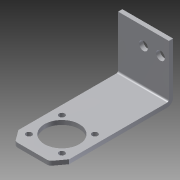
# Autodesk Inventor part: bracket for PG-71
Saved by Autodesk Inventor 2013 (Build 170138000, 138)
## iProperties
Created: 2013-02-02
Part Number: bracket for PG-71
Material: Aluminum 6061
Document SubType Name: Sheet Metal
Designer: aslane
Density: 1 g/cm^3
Sheet Metal Rule: Default
Author: aslane
Autodesk Inventor part; units mm, degrees
ref_plane "YZ Plane" through (0, 0, 0) normal (1, 0, 0) x (0, 1, 0)
ref_plane "XZ Plane" through (0, 0, 0) normal (0, 1, 0) x (-1, 0, 0)
ref_plane "XY Plane" through (0, 0, 0) normal (0, 0, 1) x (1, 0, 0)
sketch "Sketch1" plane through (0, 0, 0) normal (0, 1, 0) x (-1, 0, 0)
  line L0 (30.798, 43.1648) -> (0.6237, 2.4295)
  arc A0 (0.6237, 2.4295) -> (0, 0.5397) centre (3.175, 0.5397) ccw
  line L1 (0, 0.5397) -> (0, 0)
  line L2 (0, 0) -> (88.9, 0)
  line L3 (88.9, 0) -> (88.9, 0.5397)
  arc A1 (88.9, 0.5397) -> (88.2763, 2.4295) centre (85.725, 0.5397) ccw
  line L4 (88.2763, 2.4295) -> (58.102, 43.1648)
  arc A2 (58.102, 43.1648) -> (55.5507, 44.45) centre (55.5507, 41.275) ccw
  line L5 (55.5507, 44.45) -> (33.3493, 44.45)
  arc A3 (33.3493, 44.45) -> (30.798, 43.1648) centre (33.3493, 41.275) ccw
  circle A4 centre (15.875, 9.525) radius 4.7625
  circle A5 centre (44.45, 22.225) radius 13.0556
  circle A6 centre (56.8248, 34.5998) radius 2.1463
  circle A7 centre (56.8248, 9.8502) radius 2.1463
  circle A8 centre (32.0752, 9.8502) radius 2.1463
  circle A9 centre (32.0752, 34.5998) radius 2.1463
  circle A10 centre (73.025, 9.525) radius 4.7625
  line L6 (0, 0) -> (0, -42.1767)
  line L7 (0, -42.1767) -> (88.9, -42.1767)
  line L8 (88.9, -42.1767) -> (88.9, 0)
  dimension "d70" = 86.6267
  dimension "d71" = 3.175
  dimension "d72" = 9.525
  dimension "d73" = 4.2926
  dimension "d74" = 26.1112
  dimension "d75" = 143.471
  dimension "d76" = 90
  dimension "d77" = 36.529
  dimension "d78" = 90
  dimension "d79" = 88.9
  dimension "d80" = 44.45
  dimension "d81" = 88.9
  dimension "d82" = 72.3812
  dimension "d83" = 44.45
  dimension "d84" = 0.9449
  dimension "d85" = 15.875
  dimension "d86" = 8.0319
  dimension "d87" = 32.0752
  dimension "d88" = 6.1244
  dimension "d89" = 32.0752
  dimension "d90" = 20.8561
  dimension "d91" = 44.45
  dimension "d92" = 23.4341
  dimension "d93" = 56.8248
  dimension "d94" = 26.0121
  dimension "d95" = 56.8248
  dimension "d96" = 40.7438
  dimension "d97" = 73.025
  dimension "d98" = 53.9552
  measures "d70" distance between parallel lines of L7 L5
  measures "d71" radius of A1
  measures "d72" diameter of A10
  measures "d73" diameter of A6
  measures "d74" diameter of A5
  measures "d75" angle of L3 L4
  measures "d76" angle of L3 L5
  measures "d77" angle of L3 L0
  measures "d78" angle of L5 L1
  measures "d79" distance between parallel lines of L8 L6
  measures "d80" distance between parallel lines of L2 L5
  measures "d81" distance from line of point (0, 0) L3
  measures "d82" distance from line of point (0, 0) L4
  measures "d83" distance from line of point (0, 0) L5
  measures "d84" distance from line of point (0, 0) L0
  measures "d85" distance from line of A10.centre L3
  measures "d86" distance from line of A10.centre L4
  measures "d87" distance from line of A6.centre L3
  measures "d88" distance from line of A6.centre L4
  measures "d89" distance from line of A7.centre L3
  measures "d90" distance from line of A7.centre L4
  measures "d91" distance from line of A5.centre L3
  measures "d92" distance from line of A5.centre L4
  measures "d93" distance from line of A9.centre L3
  measures "d94" distance from line of A9.centre L4
  measures "d95" distance from line of A8.centre L3
  measures "d96" distance from line of A8.centre L4
  measures "d97" distance from line of A4.centre L3
  measures "d98" distance from line of A4.centre L4
extrude "Plate1" add sketch "Sketch1" along normal blind 3.175
sketch "Sketch9" plane through (-88.9, 0, -39.0017) normal (0, 0, -1) x (-1, 0, 0)
  line L0 (-88.9, 0) -> (0, 0)
  line L1 (0, 0) -> (0, 37.465)
  line L2 (0, 37.465) -> (-88.9, 37.465)
  line L3 (-88.9, 37.465) -> (-88.9, 0)
  constraints: 6 end point, 1 horizontal, 1 perpendicular, 1 vertical
edge flange "Flange2" height 37.465 angle 90 thickness 3.175 bend radius 1.27 thickness toward (0, 0, -1) relief straight relief width 3.175 relief depth 1.5875 edges at (-44.45, 3.175, -42.1767) wall of the first edge with corners at (0, 0, -39.0017) (-88.9, 0, -39.0017) (-88.9, 37.465, -39.0017) (0, 37.465, -39.0017)
bend "Bend5"
corner "Corner2"
sketch "Sketch10" plane through (-88.9, 37.465, -42.1767) normal (0, 1, 0) x (1, 0, 0)
  line L0 (88.9, 0) -> (0, 0) projected
  line L1 (0, -3.175) -> (0, 0) projected
  line L2 (88.9, -3.175) -> (0, -3.175) projected
  line L3 (88.9, -3.175) -> (88.9, 0) projected
  point P0 (88.9, -42.1767)
extrude "Extrusion1" add sketch "Sketch10" along normal blind 5.2324
sketch "Sketch12" plane through (0, 3.175, 0) normal (0, 1, 0) x (1, 0, 0)
  line L0 (0, 37.7317) -> (-88.9, 37.7317) projected
  arc A0 (-88.9, -0.5397) -> (-88.2763, -2.4295) centre (-85.725, -0.5397) ccw projected
  line L1 (-58.102, -43.1648) -> (-88.2763, -2.4295) projected
  line L2 (-0.6237, -2.4295) -> (-30.798, -43.1648) projected
  arc A1 (-0.6237, -2.4295) -> (0, -0.5397) centre (-3.175, -0.5397) ccw projected
  line L3 (0, 37.7317) -> (0, -0.5397) projected
  circle A2 centre (-73.025, -9.525) radius 4.7625 projected
  circle A3 centre (-15.875, -9.525) radius 4.7625 projected
  line L4 (-88.9, -0.5397) -> (-63.5, -0.5397)
  line L5 (-63.5, -0.5397) -> (-63.5, -35.8775)
  line L6 (-63.5, -0.5397) -> (-63.5, 40.7353)
  line L7 (-63.5, 40.7353) -> (-88.9, 40.7353)
  line L8 (-88.9, 40.7353) -> (-88.9, -0.5397)
  line L9 (0, 37.7317) -> (-25.4, 37.7317)
  line L10 (-25.4, 37.7317) -> (-25.4, 44.0817)
  line L11 (-25.4, 44.0817) -> (0, 44.0817)
  line L12 (0, 44.0817) -> (0, 32.5123)
  line L13 (-25.4, 37.7317) -> (-25.4, -35.8775)
  line L14 (-33.3493, -44.45) -> (-55.5507, -44.45) projected
  line L15 (-88.9, 37.7317) -> (-88.9, 47.3418)
  line L16 (-88.9, 47.3418) -> (-63.5, 47.3418)
  line L17 (-63.5, 47.3418) -> (-63.5, 37.7317)
  point P0 (0, 0)
  dimension "d64" = 25.4
  dimension "d65" = 41.275
  dimension "d66" = 25.4
  dimension "d67" = 6.35
  constraints: 26 end point, 7 perpendicular, 6 point on line, 2 parallel, 1 collinear, 1 tangent
  measures "d64" distance of L4.start L4.end
  measures "d65" distance of L4.end L6.end
  measures "d66" distance of L0.start L9.end
  measures "d67" distance of L9.end L10.end
extrude "Extrusion3" cut sketch "Sketch12" along normal mid plane 56438.8
sketch "Sketch13" plane through (-63.5, 42.6974, -39.0017) normal (0, 0, 1) x (1, 0, 0)
  ellipse E0 centre (-29.9888, -12.7) end of major axis (-29.9888, -9.398) minor radius 2.2327 projected
  ellipse E1 centre (-21.4017, -12.7) end of major axis (-21.4017, -9.398) minor radius 2.2327 projected
  point P0 (63.5, -42.6974)
  constraints: 2 other
extrude "Cut4" cut sketch "Sketch13" against normal blind 3.175
equation "\"d101\" = Thickness"
equation "\"d52\" = BendReliefWidth"
equation "\"d53\" = BendReliefDepth"
equation "\"d54\" = MinimumRemnant"
equation "\"d55\" = BendRadius"
equation "\"d59\" = CornerReliefSize"
equation "\"d60\" = GapSize"
equation "\"d61\" = JacobiRadiusSize"
equation "\"BendRadius\" = Thickness"
equation "\"BendReliefWidth\" = Thickness"
equation "\"BendReliefDepth\" = 0.5 * Thickness"
equation "\"CornerReliefSize\" = 4 * Thickness"
equation "\"MinimumRemnant\" = 2 * Thickness"
equation "\"TransitionRadius\" = BendRadius"
equation "\"JacobiRadiusSize\" = BendRadius"
equation "\"GapSize\" = Thickness"
equation "\"d1\" = BendRadius"
equation "\"Thickness\" = 3.175"
body "Solid1"
